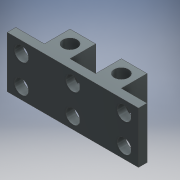
# Autodesk Inventor part: chassiconnector
Saved by Autodesk Inventor 2016 (Build 200138000, 138)
## iProperties
Created: 2017-01-05
Part Number: chassiconnector
Material: Generic
Document SubType Name: Modeling
Designer: hesaon
Density: 1 g/cm^3
Appearance: Default
Author: hesaon
Autodesk Inventor part; units mm, degrees
ref_plane "YZ Plane" through (0, 0, 0) normal (1, 0, 0) x (0, 1, 0)
ref_plane "XZ Plane" through (0, 0, 0) normal (0, 1, 0) x (-1, 0, 0)
ref_plane "XY Plane" through (0, 0, 0) normal (0, 0, 1) x (1, 0, 0)
sketch "Sketch1" plane through (0, 0, 0) normal (0, 1, 0) x (-1, 0, 0)
  line L0 (0, 0) -> (46, 0)
  line L1 (46, 0) -> (46, -18)
  line L2 (46, -18) -> (0, -18)
  line L3 (0, -18) -> (0, 0)
  circle A0 centre (41, -4) radius 2.5
  circle A1 centre (41, -14) radius 2.5
  circle A2 centre (5, -4) radius 2.5
  circle A3 centre (5, -14) radius 2.5
  circle A4 centre (23, -4) radius 2.5
  circle A5 centre (23, -14) radius 2.5
  dimension "d0" = 46
  dimension "d1" = 18
  dimension "d2" = 5
  dimension "d3" = 5
  dimension "d4" = 4
  dimension "d5" = 5
  dimension "d6" = 5
  dimension "d7" = 5
  dimension "d8" = 10
  dimension "d9" = 5
  dimension "d10" = 10
  dimension "d13" = 5
  dimension "d14" = 5
  dimension "d15" = 18
  dimension "d16" = 18
  constraints: 8 end point, 6 centre point, 4 horizontal alignment, 2 parallel, 1 horizontal, 1 perpendicular, 1 vertical alignment
  measures "d0" distance of L1.end L2.end
  measures "d1" distance of L0.end L1.end
  measures "d2" diameter of A0
  measures "d3" distance from line of A0.centre L1
  measures "d4" distance from line of L0 A0.centre
  measures "d5" diameter of A1
  measures "d6" diameter of A2
  measures "d7" distance from line of L3 A2.centre
  measures "d8" distance of A0.centre A1.centre
  measures "d9" diameter of A3
  measures "d10" distance of A3.centre A2.centre
  measures "d13" diameter of A4
  measures "d14" diameter of A5
  measures "d15" distance of A4.centre A0.centre
  measures "d16" distance of A1.centre A5.centre
extrude "Extrusion2" add sketch "Sketch1" along normal blind 3
sketch "Sketch3" plane through (0, 3, 0) normal (0, 1, 0) x (1, 0, 0)
  line L0 (-46, 0) -> (0, 0) projected
  line L1 (-46, 18) -> (0, 18) projected
  line L2 (-36, 0) -> (-27, 0)
  line L3 (-27, 0) -> (-27, 18)
  line L4 (-27, 18) -> (-36, 18)
  line L5 (-36, 18) -> (-36, 0)
  line L6 (-18, 0) -> (-9, 0)
  line L7 (-9, 0) -> (-9, 18)
  line L8 (-9, 18) -> (-18, 18)
  line L9 (-18, 18) -> (-18, 0)
  dimension "d19" = 9
  dimension "d20" = 9
  dimension "d21" = 9
  dimension "d22" = 9
  constraints: 16 end point, 4 parallel, 4 point on line, 2 horizontal, 2 perpendicular
  measures "d19" distance of L4.end L3.end
  measures "d20" distance between parallel lines of L7 L9
  measures "d21" distance of L0.end L6.end
  measures "d22" distance of L6.start L2.end
extrude "Extrusion3" add sketch "Sketch3" along normal blind 9 contours L5 L1 L3 L0 | L9 L1 L7 L0
hole "Hole1" at (-31.5, 7.5, 0) direction (0, 0, -1) diameter 5 end through all
hole "Hole2" at (-13.5, 7.5, 0) direction (0, 0, -1) diameter 5 end through all
sketch "Sketch4" plane through (0, 0, -18) normal (0, 0, -1) x (-1, 0, 0)
  line L0 (9, 3) -> (9, 12) projected
  line L1 (18, 3) -> (18, 12) projected
  line L2 (9, 12) -> (18, 12)
  line L3 (18, 12) -> (18, 3)
  line L4 (18, 3) -> (9, 3)
  line L5 (9, 3) -> (9, 12)
  line L6 (27, 3) -> (27, 12) projected
  line L7 (36, 3) -> (46, 3) projected
  line L8 (27, 12) -> (36, 12)
  line L9 (36, 12) -> (36, 3)
  line L10 (36, 3) -> (27, 3)
  line L11 (27, 3) -> (27, 12)
  point P0 (0, 0)
  constraints: 16 end point, 4 parallel, 2 horizontal, 2 perpendicular
extrude "Extrusion4" cut sketch "Sketch4" against normal blind 9
body "Solid2"
